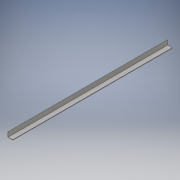
# Autodesk Inventor part: 32 L bracket
Saved by Autodesk Inventor 2016 SP2 (Build 200236200, 236)
## iProperties
Created: 2018-01-17
Part Number: 32 L bracket
Material: Generic
Document SubType Name: Modeling
Designer: CAD
Density: 1 g/cm^3
Appearance: Default
Author: CAD
Autodesk Inventor part; units mm, degrees
ref_plane "YZ Plane" through (0, 0, 0) normal (1, 0, 0) x (0, 1, 0)
ref_plane "XZ Plane" through (0, 0, 0) normal (0, 1, 0) x (-1, 0, 0)
ref_plane "XY Plane" through (0, 0, 0) normal (0, 0, 1) x (1, 0, 0)
sketch "Sketch1" plane through (0, 0, 0) normal (0, 0, 1) x (1, 0, 0)
  line L0 (0, 0) -> (0, 25.4)
  line L1 (0, 0) -> (25.4, 0)
  line L2 (25.4, 3.175) -> (3.175, 3.175)
  line L3 (3.175, 3.175) -> (3.175, 25.4)
  line L4 (25.4, 3.175) -> (25.4, 0)
  line L5 (0, 25.4) -> (3.175, 25.4)
  dimension "d0" = 25.4
  dimension "d1" = 25.4
  dimension "d2" = 3.175
  constraints: 12 end point, 2 horizontal, 2 vertical, 1 other
  measures "d0" distance of L0.start L0.end
  measures "d1" distance of L0.start L1.end
  measures "d2" distance between parallel lines of L1 L2
extrude "Extrusion1" add sketch "Sketch1" along normal blind 812.8
body "Solid1"
